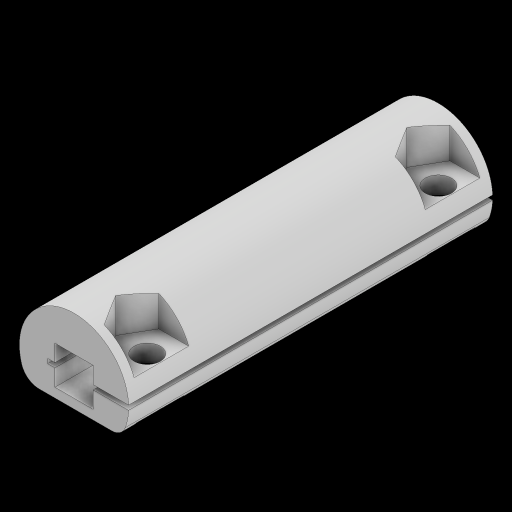
# Autodesk Inventor part: AxleBar
Saved by Autodesk Inventor 2024.1 (Build 281209000, 209)
## iProperties
Created: 2025-01-21
Part Number: AxleBar
Material: Generic
Document SubType Name: Modeling
Designer: Teddy
Density: 1 g/cm^3
Appearance: Default
Author: Teddy
Autodesk Inventor part; units mm, degrees
ref_plane "YZ Plane" through (0, 0, 0) normal (1, 0, 0) x (0, 1, 0)
sketch "Sketch1" plane through (0, 0, 0) normal (0, 0, 1) x (1, 0, 0)
  line L0 (-3.3274, -3.3274) -> (3.3274, -3.3274)
  line L1 (3.3274, -3.3274) -> (3.3274, 3.3274)
  line L2 (3.3274, 3.3274) -> (-3.3274, 3.3274)
  line L3 (-3.3274, 3.3274) -> (-3.3274, -3.3274)
  line L4 (-3.3274, -3.3274) -> (3.3274, 3.3274) construction
  line L5 (3.3274, -3.3274) -> (-3.3274, 3.3274) construction
  circle A0 centre (0, 0) radius 9.525
  line L6 (-4.5974, 0.3969) -> (11.7358, 0.3969)
  line L7 (11.7358, 0.3969) -> (11.7358, -0.3969)
  line L8 (11.7358, -0.3969) -> (-4.5974, -0.3969)
  line L9 (-4.5974, -0.3969) -> (-4.5974, 0.3969)
  point P0 (-4.5974, 0)
  point P1 (-3.3274, -0.3969)
  point P2 (-3.3274, 0.3969)
  point P3 (3.3274, 0.3969)
  point P4 (9.5167, 0.3969)
  point P5 (9.5167, -0.3969)
  point P6 (3.3274, -0.3969)
  dimension "d0" = 6.6548
  dimension "d1" = 6.6548
  dimension "d2" = 19.05
  dimension "d3" = 0.7937
  dimension "d4" = 1.27
  constraints: 20 end point, 4 parallel, 3 midpoint, 2 horizontal, 2 perpendicular, 1 centre point, 1 coincident, 1 horizontal alignment
  measures "d0" distance between parallel lines of L2 L0
  measures "d1" distance between parallel lines of L3 L1
  measures "d2" diameter of A0
  measures "d3" distance between parallel lines of L6 L8
  measures "d4" distance between parallel lines of L3 L9
extrude "Extrusion1" add sketch "Sketch1" along normal blind 63.5 contours L0 L1 L8 A0 L6 L2 L3 L9
sketch "Sketch2" plane through (3.3274, 0.3969, 0) normal (0, -1, 0) x (1, 0, 0)
  circle A0 centre (3.0947, 57.15) radius 2.286
  line L0 (0, 63.5) -> (6.1893, 63.5) projected
  line L1 (6.1893, 0) -> (6.1893, 63.5) projected
  line L2 (6.1893, 31.75) -> (0, 31.75)
  line L3 (0, 0) -> (0, 63.5) projected
  circle A1 centre (3.0947, 6.35) radius 2.286
  point P0 (-3.3274, 0)
  point P1 (3.0947, 63.5)
  dimension "d7" = 4.572
  dimension "d8" = 6.35
  constraints: 3 midpoint, 2 centre point, 2 end point, 1 symmetric about line, 1 vertical alignment, 1 other
  measures "d7" diameter of A0
  measures "d8" distance from line of L0 A0.centre
extrude "Extrusion2" cut sketch "Sketch2" along normal mid plane 63.5 contours A0 | A1
ref_plane "Work Plane1" through (0, -9.525, 0) normal (0, -1, 0) x (1, 0, 0)
ref_plane "Work Plane2" through (0, 9.525, 0) normal (0, 1, 0) x (1, 0, 0)
sketch "Sketch3" plane through (0, -9.525, 0) normal (0, -1, 0) x (1, 0, 0)
  circle A0 centre (6.4221, 6.35) radius 2.286 projected
  circle A1 centre (6.4221, 6.35) radius 4.1275
  line L0 (6.4221, 10.4775) -> (9.5167, 10.4775)
  line L1 (9.5167, 0) -> (9.5167, 63.5) projected
  line L2 (6.4221, 2.2225) -> (9.5167, 2.2225)
  line L3 (-9.525, 0) -> (-9.525, 63.5) projected
  line L4 (-9.525, 31.75) -> (9.5167, 31.75)
  circle A2 centre (6.4221, 57.15) radius 4.1275
  line L5 (6.4221, 53.0225) -> (9.5167, 53.0225)
  line L6 (6.4221, 61.2775) -> (9.5167, 61.2775)
  point P0 (0, 0)
  dimension "d11" = 8.255
  constraints: 10 end point, 5 symmetric about line, 4 point on circle, 2 centre point, 2 horizontal, 2 point on line, 1 coincident, 1 midpoint, 1 parallel, 1 tangent, 1 other
  measures "d11" diameter of A1
extrude "Extrusion3" cut sketch "Sketch3" against normal blind 5.715 contours A1 L1 | L0 L1 A1 | A1 L1 L2 | L5 A2 L1 | A2 L1 | A2 L6 L1 picked at (9.2472, 6.35) picked at (7.5728, 58.1798)
sketch "Sketch4" plane through (0, 9.525, 0) normal (0, 1, 0) x (1, 0, 0)
  circle A0 centre (6.4221, -6.35) radius 2.286 projected
  arc A1 (6.4221, -2.2225) -> (6.4221, -10.4775) centre (6.4221, -6.35) ccw projected
  line L0 (0.9228, -6.35) -> (3.6724, -1.5875)
  line L1 (3.6724, -1.5875) -> (9.1717, -1.5875)
  line L2 (9.1717, -1.5875) -> (11.9213, -6.35)
  line L3 (11.9213, -6.35) -> (9.1717, -11.1125)
  line L4 (9.1717, -11.1125) -> (3.6724, -11.1125)
  line L5 (3.6724, -11.1125) -> (0.9228, -6.35)
  line L6 (-9.525, 0) -> (-9.525, -63.5) projected
  line L7 (-9.525, -31.75) -> (9.525, -31.75)
  line L8 (9.1717, -11.1125) -> (11.7374, -11.1125)
  line L9 (11.7374, -11.1125) -> (11.7374, -1.5875)
  line L10 (11.7374, -1.5875) -> (9.1717, -1.5875)
  line L11 (0.9228, -57.15) -> (3.6724, -61.9125)
  line L12 (3.6724, -61.9125) -> (9.1717, -61.9125)
  line L13 (9.1717, -61.9125) -> (11.9213, -57.15)
  line L14 (11.9213, -57.15) -> (9.1717, -52.3875)
  line L15 (9.1717, -52.3875) -> (3.6724, -52.3875)
  line L16 (3.6724, -52.3875) -> (0.9228, -57.15)
  line L17 (9.1717, -52.3875) -> (11.7374, -52.3875)
  line L18 (11.7374, -52.3875) -> (11.7374, -61.9125)
  line L19 (11.7374, -61.9125) -> (9.1717, -61.9125)
  point P0 (0, 0)
  point P1 (11.7374, -6.6685)
  point P2 (11.7374, -6.0315)
  dimension "d16" = 9.525
  constraints: 38 end point, 8 symmetric about line, 2 horizontal, 2 perpendicular, 1 coincident, 1 midpoint, 13 other
  measures "d16" distance between parallel lines of L4 L1
extrude "Extrusion4" cut sketch "Sketch4" against normal blind 6.096 contours A0 | L0 L1 L2 L9 L3 L4 L5 | L10 L9 L2 | L3 L9 L8 | L16 L15 L14 L18 L13 L12 L11 | L13 L18 L19 | L17 L18 L14
sketch "Sketch5" plane through (0, 0, 63.5) normal (0, 0, 1) x (1, 0, 0)
  line L0 (4.1361, -3.81) -> (8.7081, -3.81) projected
  arc A0 (9.5167, 0.3969) -> (9.5167, -0.3969) centre (0, 0) ccw projected
  line L1 (8.1359, -4.953) -> (-8.1359, -4.953)
  arc A1 (-8.1359, -4.953) -> (8.1359, -4.953) centre (0, 0) ccw
  dimension "d17" = 1.143
  constraints: 4 point on circle, 2 end point, 1 centre point, 1 coincident, 1 horizontal
  measures "d17" distance between parallel lines of L0 L1
extrude "Extrusion5" cut sketch "Sketch5" against normal up to surface (63.5 mm away)
fillet "Fillet1" radius 3.175 1 edges at (-8.1359, -4.953, 31.75)
fillet "Fillet2" radius 2.54 3 edges at (8.1359, -4.953, 31.75) (8.1359, -4.953, 62.3888) (8.1359, -4.953, 1.1112)
body "Solid1"
